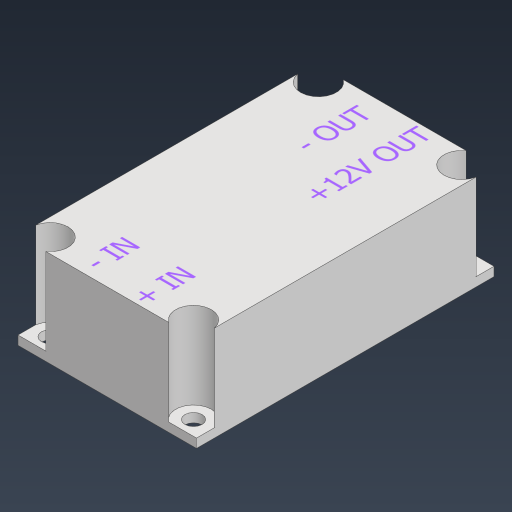
# Autodesk Inventor part: led_buck_conv
Saved by Autodesk Inventor 2023 (Build 270158000, 158)
## iProperties
Created: 2025-12-26
Part Number: led_buck_conv
Material: Generic
Document SubType Name: Modeling
Designer: szymo
Density: 1 g/cm^3
Appearance: Default
Author: szymo
Autodesk Inventor part; units mm, degrees
ref_plane "YZ Plane" through (0, 0, 0) normal (1, 0, 0) x (0, 1, 0)
ref_plane "XZ Plane" through (0, 0, 0) normal (0, 1, 0) x (-1, 0, 0)
ref_plane "XY Plane" through (0, 0, 0) normal (0, 0, 1) x (1, 0, 0)
sketch "Sketch1" plane through (0, 0, 0) normal (0, 1, 0) x (-1, 0, 0)
  line L0 (0, 0) -> (-30, 0)
  line L1 (-30, 0) -> (-30, -50)
  line L2 (-30, -50) -> (0, -50)
  line L3 (0, -50) -> (0, 0)
  circle A0 centre (-2.95, -2.45) radius 1.45
  circle A1 centre (-2.95, -47.55) radius 1.45
  circle A2 centre (-27.05, -2.45) radius 1.45
  circle A3 centre (-27.05, -47.55) radius 1.45
  dimension "d0" = 30
  dimension "d1" = 50
  dimension "d2" = 2.9
  dimension "d3" = 2.9
  dimension "d4" = 2.9
  dimension "d5" = 2.9
  dimension "d6" = 1
  dimension "d7" = 1
  dimension "d8" = 1.5
  dimension "d9" = 1.5
  dimension "d10" = 21.2
  dimension "d11" = 1
  dimension "d12" = 1
  dimension "d13" = 1.5
  dimension "d14" = 1.5
  dimension "d15" = 21.2
  dimension "d16" = 42.2
  constraints: 8 end point, 4 centre point, 2 parallel, 1 horizontal, 1 perpendicular
  measures "d0" distance of L2.end L1.end
  measures "d1" distance of L1.end L0.end
  measures "d2" diameter of A0
  measures "d3" diameter of A2
  measures "d4" diameter of A3
  measures "d5" diameter of A1
  measures "d6" distance edge to line of A0 L0
  measures "d7" distance edge to line of A2 L0
  measures "d8" distance edge to line of A0 L3
  measures "d9" distance edge to line of A2 L1
  measures "d11" distance edge to line of A1 L2
  measures "d12" distance edge to line of A3 L2
  measures "d13" distance edge to line of A3 L1
  measures "d14" distance edge to line of A1 L3
extrude "Extrusion1" add sketch "Sketch1" along normal blind 1.5
sketch "Sketch2" plane through (0, 0, 0) normal (0, 1, 0) x (-1, 0, 0)
  line L0 (-30, 0) -> (-30, -50) projected
  line L1 (-30, -50) -> (0, -50) projected
  line L2 (0, -50) -> (0, 0) projected
  line L3 (0, 0) -> (-30, 0) projected
  circle A0 centre (-2.95, -2.45) radius 1.45 projected
  circle A1 centre (-2.95, -47.55) radius 1.45 projected
  circle A2 centre (-27.05, -2.45) radius 1.45 projected
  circle A3 centre (-27.05, -47.55) radius 1.45 projected
  circle A4 centre (-2.95, -2.45) radius 3
  circle A5 centre (-27.05, -2.45) radius 3
  circle A6 centre (-27.05, -47.55) radius 3
  circle A7 centre (-2.95, -47.55) radius 3
  point P0 (-4.6813, -50)
  point P1 (0, -47.0046)
  point P2 (0, -2.9954)
  point P3 (-4.6813, 0)
  point P4 (-25.3187, 0)
  point P5 (-30, -2.9954)
  point P6 (-30, -47.0046)
  point P7 (-25.3187, -50)
  dimension "d19" = 6
  dimension "d20" = 6
  dimension "d21" = 6
  dimension "d22" = 6
  constraints: 4 centre point, 4 coincident
  measures "d19" diameter of A4
  measures "d20" diameter of A5
  measures "d21" diameter of A6
  measures "d22" diameter of A7
extrude "Extrusion2" add sketch "Sketch2" along normal blind 16 contours A5 L3 A4 L2 A7 L1 A6 L0
sketch "Sketch3" plane through (0, 16, 0) normal (0, 1, 0) x (1, 0, 0)
  line L0 (8.9716, 1.646) -> (8.9716, 8.8387) construction
  line L1 (8.9716, 8.8387) -> (12.0196, 8.8387) construction
  line L2 (12.0196, 8.8387) -> (12.0196, 1.646) construction
  line L3 (12.0196, 1.646) -> (8.9716, 1.646) construction
  line L4 (17.94, 0.53) -> (17.94, 9.2516) construction
  line L5 (17.94, 9.2516) -> (20.988, 9.2516) construction
  line L6 (20.988, 9.2516) -> (20.988, 0.53) construction
  line L7 (20.988, 0.53) -> (17.94, 0.53) construction
  line L8 (9.4001, 36.4792) -> (9.4001, 48.0764) construction
  line L9 (9.4001, 48.0764) -> (12.819, 48.0764) construction
  line L10 (12.819, 48.0764) -> (12.819, 36.4792) construction
  line L11 (12.819, 36.4792) -> (9.4001, 36.4792) construction
  line L12 (17.4365, 29.8752) -> (17.4365, 49.4772) construction
  line L13 (17.4365, 49.4772) -> (20.6129, 49.4772) construction
  line L14 (20.6129, 49.4772) -> (20.6129, 29.8752) construction
  line L15 (20.6129, 29.8752) -> (17.4365, 29.8752) construction
  dimension "d0" = 30
  dimension "d1" = 50
  dimension "d2" = 2.9
  dimension "d3" = 2.9
  dimension "d4" = 2.9
  dimension "d5" = 2.9
  dimension "d6" = 1
  dimension "d7" = 1
  dimension "d8" = 1.5
  dimension "d9" = 1.5
  dimension "d10" = 21.2
  dimension "d11" = 1
  dimension "d12" = 1
  dimension "d13" = 1.5
  dimension "d14" = 1.5
  dimension "d15" = 21.2
  dimension "d16" = 42.2
  constraints: 8 other
equation "\"d3\" = d2"
equation "\"d4\" = d2"
equation "\"d5\" = d2"
equation "\"d7\" = d6"
equation "\"d12\" = d11"
body "Solid1"
